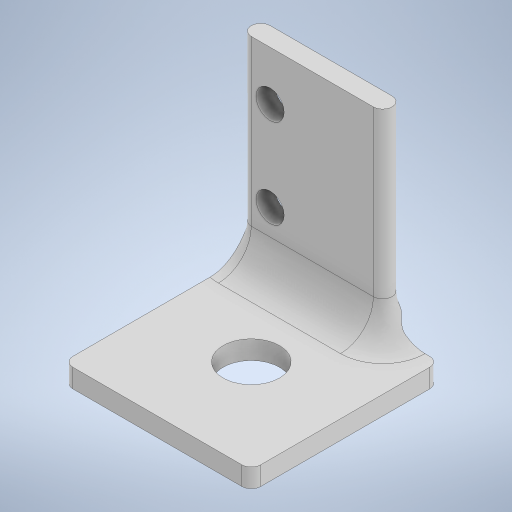
# Autodesk Inventor part: LimitSwitch Mount
Saved by Autodesk Inventor 2023.2 (Build 272271030, 271C)
## iProperties
Created: 2023-04-27
Part Number: LimitSwitch Mount
Material: Generic
Document SubType Name: Modeling
Designer: ethan
Density: 1 g/cm^3
Appearance: Default
Author: ethan
Autodesk Inventor part; units mm, degrees
ref_plane "YZ Plane" through (0, 0, 0) normal (1, 0, 0) x (0, 1, 0)
ref_plane "XZ Plane" through (0, 0, 0) normal (0, 1, 0) x (-1, 0, 0)
ref_plane "XY Plane" through (0, 0, 0) normal (0, 0, 1) x (1, 0, 0)
sketch "Sketch1" plane through (0, 0, 0) normal (0, 0, 1) x (1, 0, 0)
  line L0 (0, 0) -> (-20, 0)
  line L1 (-20, 0) -> (-20, 25)
  line L2 (-20, 25) -> (0, 25)
  line L3 (0, 25) -> (0, 0)
  circle A0 centre (-17, 19.75) radius 1.5
  circle A1 centre (-17, 10.25) radius 1.5
  line L4 (-17, 19.75) -> (-17, 10.25) construction
  line L5 (-20, 0) -> (0, 0)
  line L6 (0, 0) -> (0, 2)
  line L7 (0, 2) -> (-20, 2)
  line L8 (-20, 2) -> (-20, 0)
  line L9 (-5, 25) -> (-5, 2)
  dimension "d0" = 20
  dimension "d1" = 25
  dimension "d7" = 3
  dimension "d8" = 3
  dimension "d9" = 9.5
  dimension "d10" = 17
  dimension "d11" = 5.25
  dimension "d15" = 2
  dimension "d22" = 15
  constraints: 20 end point, 4 parallel, 3 perpendicular, 3 point on line, 2 centre point, 2 horizontal, 1 vertical
  measures "d0" distance of L1.end L2.end
  measures "d1" distance of L0.end L1.end
  measures "d7" diameter of A0
  measures "d8" diameter of A1
  measures "d9" distance of L4.end L4.start
  measures "d10" distance from line of L3 L4.start
  measures "d11" distance from line of L2 L4.start
  measures "d15" distance of L6.end L5.end
  measures "d22" distance between parallel lines of L9 L1
extrude "Extrusion1" add sketch "Sketch1" along normal blind 2 contours L1 L2 L9 L7
sketch "Sketch4" plane through (-20, 2, 0) normal (0, -1, 0) x (1, 0, 0)
  line L0 (20, 0) -> (0, 0) projected
  line L1 (0, 0) -> (20, 0)
  line L2 (20, 0) -> (20, 21)
  line L3 (20, 21) -> (0, 21)
  line L4 (0, 21) -> (0, 0)
  line L5 (0, 1) -> (20, 1)
  line L6 (0, 21) -> (20, 1) construction
  circle A0 centre (10, 11) radius 3
  point P0 (15, 0)
  dimension "d18" = 21
  dimension "d21" = 20
  dimension "d23" = 6
  constraints: 12 end point, 2 parallel, 2 perpendicular, 2 point on line, 1 centre point, 1 coincident, 1 horizontal, 1 midpoint
  measures "d18" distance of L2.end L1.end
  measures "d21" distance between parallel lines of L3 L5
  measures "d23" diameter of A0
extrude "Extrusion4" add sketch "Sketch4" against normal blind 2 contours L5 L4 L3 L2
chamfer "Chamfer1" distance 1 angle 45 1 edges at (-5, 3, 1)
fillet "Fillet1" radius 1 10 edges at (-20, 3, 21) (0, 3, 21) (0, 3, 1) (-20, 13.5, 0) (-20, 14.5, 2) (-5, 14.5, 2) (-5, 13.5, 0) (-5, 2, 0.0001) (-5, 3, 0.0001) (-4.0001, 3, 1)
sketch "Sketch5" plane through (-20, 4, 0) normal (0, 1, 0) x (1, 0, 0)
  line L0 (1, -2) -> (14, -2) projected
  line L1 (14, -2) -> (1, -2)
  line L2 (2, -2) -> (2, -7)
  line L3 (2, -7) -> (13, -7)
  line L4 (13, -7) -> (13, -1.9771)
  point P0 (20, 0)
  point P1 (13, -2)
  dimension "d29" = 5
  dimension "d41" = 1
  dimension "d42" = 1
  constraints: 8 end point, 2 parallel, 1 horizontal, 1 perpendicular, 1 point on line
  measures "d29" distance of L2.start L2.end
  measures "d41" distance from line of L0.end L4
  measures "d42" distance from line of L2 L0.start
fillet "Fillet3" radius 3.5 3 edges at (-5, 4, 1) (-19.7071, 4, 1.7071) (-12.5, 4, 2)
body "Solid1"
